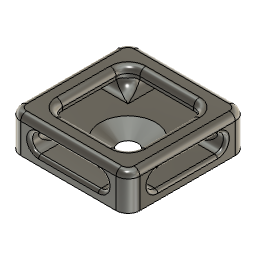
ziptiescrew (Autodesk Fusion 360 design; units mm, degrees)
Autodesk Fusion 360 part; units mm, degrees
sketch "Sketch1" plane through (0, 0, 0) normal (0, 0, 1) x (1, 0, 0)
  line L0 (0, 0) -> (20, 0)
  line L1 (20, 0) -> (20, 20)
  line L2 (20, 20) -> (0, 20)
  line L3 (0, 20) -> (0, 0)
  dimension "d1" = 20
  dimension "d2" = 20
  constraint horizontal L0
  constraint vertical L1
  constraint horizontal L2
  constraint vertical L3
  constraint coincident L0.start L3.end
  measures "d1" distance of L1.end L2.end
  measures "d2" distance of L0.end L1.end
extrude "Extrude1" add sketch "Sketch1" along normal blind 6
sketch "Sketch2" plane through (20, 0, 0) normal (1, 0, 0) x (0, 1, 0)
  line L0 (0, 0) -> (20, 0)
  line L1 (20, 0) -> (20, 6)
  line L2 (20, 6) -> (0, 6)
  line L3 (0, 6) -> (0, 0)
  line L4 (3.5, 4.5) -> (16.5, 4.5)
  line L5 (16.5, 4.5) -> (16.5, 1.5)
  line L6 (16.5, 1.5) -> (3.5, 1.5)
  line L7 (3.5, 1.5) -> (3.5, 4.5)
  dimension "d5" = 1.5
  dimension "d6" = 1.5
  dimension "d7" = 3.5
  dimension "d8" = 3.5
  constraint horizontal L4
  constraint vertical L5
  constraint horizontal L6
  constraint vertical L7
  measures "d5" distance of L2 L4
  measures "d6" distance of L0 L6
  measures "d7" distance of L1 L5
  measures "d8" distance of L3 L7
extrude "Extrude2" cut sketch "Sketch2" along normal through all and the other way blind 20 contours L4 L5 L6 L7
sketch "Sketch3" plane through (0, 0, 0) normal (0, -1, 0) x (1, 0, 0)
  line L0 (0, 0) -> (20, 0)
  line L1 (20, 0) -> (20, 6)
  line L2 (20, 6) -> (0, 6)
  line L3 (0, 6) -> (0, 0)
  line L4 (3.5, 4.5) -> (16.5, 4.5)
  line L5 (16.5, 4.5) -> (16.5, 1.5)
  line L6 (16.5, 1.5) -> (3.5, 1.5)
  line L7 (3.5, 1.5) -> (3.5, 4.5)
  dimension "d12" = 1.5
  dimension "d13" = 1.5
  dimension "d14" = 3.5
  dimension "d15" = 3.5
  constraint horizontal L4
  constraint vertical L5
  constraint horizontal L6
  constraint vertical L7
  measures "d12" distance of L2 L4
  measures "d13" distance of L0 L6
  measures "d14" distance of L3 L7
  measures "d15" distance of L1 L5
extrude "Extrude3" cut sketch "Sketch3" against normal blind 20 contours L4 L5 L6 L7
sketch "Sketch4" plane through (0, 0, 6) normal (0, 0, 1) x (-1, 0, 0)
  line L0 (0, -20) -> (0, 0)
  line L1 (0, 0) -> (-20, 0)
  line L2 (-20, 0) -> (-20, -20)
  line L3 (-20, -20) -> (0, -20)
  line L4 (-3.5, -16.5) -> (-16.5, -16.5)
  line L5 (-16.5, -16.5) -> (-16.5, -3.5)
  line L6 (-16.5, -3.5) -> (-3.5, -3.5)
  line L7 (-3.5, -3.5) -> (-3.5, -16.5)
  dimension "d18" = 3.5
  dimension "d19" = 3.5
  dimension "d20" = 3.5
  dimension "d21" = 3.5
  constraint horizontal L4
  constraint vertical L5
  constraint horizontal L6
  constraint vertical L7
  measures "d18" distance of L0 L7
  measures "d19" distance of L1 L6
  measures "d20" distance of L2 L5
  measures "d21" distance of L3 L4
extrude "Extrude4" cut sketch "Sketch4" against normal up to surface (4.5 mm away) contours L4 L5 L6 L7
sketch "Sketch5" plane through (0, 0, 0) normal (0, 0, -1) x (1, 0, 0)
  line L0 (0, 0) -> (0, -20)
  line L1 (0, -20) -> (20, -20)
  line L2 (20, -20) -> (20, 0)
  line L3 (20, 0) -> (0, 0)
  circle A0 centre (10, -10) radius 1.625
  line L4 (0, 0) -> (20, -20)
  line L5 (20, 0) -> (0, -20)
  dimension "d24" = 3.25
  constraint coincident L0.start L3.end
  constraint coincident L1.end L2.start
  constraint coincident L2.end L3.start
  constraint coincident L0.end L1.start
  constraint coincident A0.centre L5
  constraint coincident A0.centre L4
  measures "d24" diameter of A0
extrude "Extrude5" cut sketch "Sketch5" against normal blind 3 contours A0 L4 L5 | A0 L4 L5 | A0 L4 L5 | A0 L4 L5
chamfer "Chamfer1" distance 3 distance2 1.5 1 edges at (8.485, 10.5876, 1.5) measured on face at (9.9595, 17.2068, 1.5)
fillet "Fillet1" radius 2 4 edges at (3.5, 16.5, 5.25) (16.5, 16.5, 5.25) (16.5, 3.5, 5.25) (3.5, 3.5, 5.25)
fillet "Fillet2" radius 2 4 edges at (0, 0, 3) (20, 0, 3) (20, 20, 3) (0, 20, 3)
fillet "Fillet3" radius 1 1 faces at (8.5, 1.1667, 6)
fillet "Fillet4" radius 1.5 16 edges at (18.25, 3.5, 4.5) (18.25, 3.5, 1.5) (18.25, 16.5, 1.5) (18.25, 16.5, 4.5) (16.5, 18.25, 4.5) (16.5, 18.25, 1.5) (3.5, 18.25, 1.5) (3.5, 18.25, 4.5) (1.75, 16.5, 1.5) (1.75, 16.5, 4.5) (1.75, 3.5, 1.5) (1.75, 3.5, 4.5) (3.5, 1.75, 4.5) (3.5, 1.75, 1.5) (16.5, 1.75, 4.5) (16.5, 1.75, 1.5)
fillet "Fillet5" radius 2 4 edges at (16.4202, 16.4202, 2.5172) (16.4202, 3.5798, 2.5172) (3.5798, 3.5798, 2.5172) (3.5798, 16.4202, 2.5172)
fillet "Fillet6" radius 0.5 16 edges at (0, 16.5, 3) (0, 10, 4.5) (0, 3.5, 3) (0, 10, 1.5) (16.5, 20, 3) (10, 20, 4.5) (3.5, 20, 3) (10, 20, 1.5) (20, 3.5, 3) (20, 10, 4.5) (20, 16.5, 3) (20, 10, 1.5) (3.5, 0, 3) (10, 0, 4.5) (16.5, 0, 3) (10, 0, 1.5)
